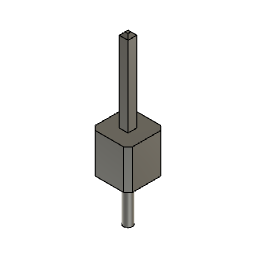
pinHeader_2.54mmp_1pin_Vertical (Autodesk Fusion 360 design; units mm, degrees)
Autodesk Fusion 360 part; units mm, degrees
sketch "スケッチ1" plane through (0, 0, 0) normal (0, 0, 1) x (1, 0, 0)
  line L0 (0, 0) -> (2.54, 0)
  line L1 (2.54, 0) -> (2.54, 2.54)
  line L2 (2.54, 2.54) -> (0, 2.54)
  line L3 (0, 2.54) -> (0, 0)
  circle A0 centre (1.27, 1.27) radius 0.3
  dimension "d1" = 2.54
  dimension "d2" = 2.54
  dimension "d12" = 0.6
  dimension "d13" = 1.27
  dimension "d14" = 1.27
  constraint horizontal L0
  constraint vertical L1
  constraint horizontal L2
  constraint vertical L3
  constraint coincident L0.start L3.end
  measures "d1" distance of L0.start L0.end
  measures "d2" distance of L0.start L2.end
  measures "d12" diameter of A0
  measures "d13" distance of L0 A0.centre
  measures "d14" distance of L3 A0.centre
extrude "押し出し1" add sketch "スケッチ1" along normal blind 2.7 contours L0 L1 L2 L3 | A0
sketch "スケッチ2" plane through (0, 0, 2.7) normal (0, 0, 1) x (-1, 0, 0)
  line L0 (0, -2.54) -> (0, 0)
  line L1 (0, 0) -> (-2.54, 0)
  line L2 (-2.54, 0) -> (-2.54, -2.54)
  line L3 (-2.54, -2.54) -> (0, -2.54)
  line L4 (-0.97, -1.57) -> (-1.57, -1.57)
  line L5 (-1.57, -1.57) -> (-1.57, -0.97)
  line L6 (-1.57, -0.97) -> (-0.97, -0.97)
  line L7 (-0.97, -0.97) -> (-0.97, -1.57)
  dimension "d5" = 0.6
  dimension "d6" = 0.6
  dimension "d7" = 0.97
  dimension "d8" = 0.97
  constraint horizontal L4
  constraint vertical L5
  constraint horizontal L6
  constraint vertical L7
  measures "d5" distance of L4.start L4.end
  measures "d6" distance of L4.start L6.end
  measures "d7" distance of L0 L7
  measures "d8" distance of L1 L6
extrude "押し出し2" add sketch "スケッチ2" along normal blind 5.7 contours L4 L5 L6 L7
chamfer "面取り1" distance 0.2 angle 45 4 edges at (1.27, 0.97, 8.4) (1.57, 1.27, 8.4) (1.27, 1.57, 8.4) (0.97, 1.27, 8.4)
extrude "押し出し3" add sketch "スケッチ1" against normal blind 3 contours A0
chamfer "面取り2" distance 0.3 angle 45 4 edges at (0, 2.54, 1.35) (0, 0, 1.35) (2.54, 0, 1.35) (2.54, 2.54, 1.35)
